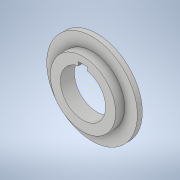
# Autodesk Inventor part: SprocketAdapter
Saved by Autodesk Inventor 2021 (Build 250183000, 183)
## iProperties
Created: 2020-09-20
Part Number: SprocketAdapter
Material: Generic
Document SubType Name: Modeling
Designer: PhotonUser
Density: 1 g/cm^3
Appearance: Default
Mass: 13.5175 g
Surface Area: 73.571 cm^2
Volume: 13.5175 cm^3
Author: PhotonUser
Autodesk Inventor part; units mm, degrees
ref_plane "YZ Plane" through (0, 0, 0) normal (1, 0, 0) x (0, 1, 0)
ref_plane "XZ Plane" through (0, 0, 0) normal (0, 1, 0) x (-1, 0, 0)
ref_plane "XY Plane" through (0, 0, 0) normal (0, 0, 1) x (1, 0, 0)
sketch "Sketch1" plane through (0, 0, 0) normal (1, 0, 0) x (0, 1, 0)
  line L0 (0, 0) -> (22.86, 0)
  line L1 (22.86, 0) -> (22.86, -6.35)
  line L2 (22.86, -6.35) -> (31.75, -6.35)
  line L3 (31.75, -6.35) -> (31.75, -9.8298)
  line L4 (31.75, -9.8298) -> (0, -9.8298)
  line L5 (0, -9.8298) -> (0, 0)
  dimension "d0" = 22.86
  dimension "d1" = 6.35
  dimension "d2" = 8.89
  dimension "d3" = 3.4798
  constraints: 12 end point, 3 perpendicular, 2 horizontal, 1 vertical
  measures "d0" distance of L0.start L0.end
  measures "d1" distance of L0.end L1.end
  measures "d2" distance of L1.end L2.end
  measures "d3" distance of L2.end L3.end
revolve "Revolution1" add sketch "Sketch1" angle 360 about axis through (0, 0, -9.8298) along (0, 0, 1)
sketch "Sketch2" plane through (0, 0, 0) normal (0, 0, 1) x (1, 0, 0)
  circle A0 centre (0, 0) radius 15.875
  line L0 (-3.175, 15.5543) -> (-3.175, 18.0943)
  line L1 (-3.175, 18.0943) -> (3.175, 18.0943)
  line L2 (3.175, 18.0943) -> (3.175, 15.5543)
  line L3 (0, 0) -> (0, 24.2947)
  point P0 (0, 0)
  point P1 (0, 18.0943)
  dimension "d5" = 31.75
  dimension "d6" = 6.35
  dimension "d7" = 2.54
  constraints: 8 end point, 2 perpendicular, 2 point on circle, 2 vertical, 1 centre point, 1 coincident, 1 midpoint, 1 point on line
  measures "d5" diameter of A0
  measures "d6" distance of L0.end L1.end
  measures "d7" distance from line of L1 L0.start
extrude "Extrusion1" cut sketch "Sketch2" against normal through all
sketch "Sketch3" plane through (0, 0, -6.35) normal (0, 0, 1) x (1, 0, 0)
  point P0 (0, 0)
body "Solid1"
